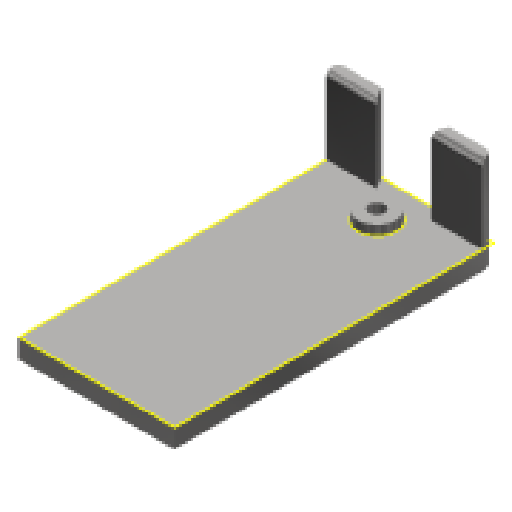
# Autodesk Inventor part: Gehäuse
Saved by Autodesk Inventor 2023 (Build 270158000, 158)
## iProperties
Created: 2025-01-24
Part Number: Gehäuse
Material: 1.2067 100 Cr 6 (WS)
Document SubType Name: Modeling
Designer: abdel
Density: 7.84 g/cm^3
Appearance: Stahl - poliert
Author: abdel
Autodesk Inventor part; units mm, degrees
ref_plane "YZ Plane" through (0, 0, 0) normal (1, 0, 0) x (0, 1, 0)
ref_plane "XZ Plane" through (0, 0, 0) normal (0, 1, 0) x (-1, 0, 0)
ref_plane "XY Plane" through (0, 0, 0) normal (0, 0, 1) x (1, 0, 0)
sketch "Skizze1" plane through (0, 0, 0) normal (0, 0, 1) x (1, 0, 0)
  line L0 (-20, 15) -> (20, 15)
  line L1 (20, 15) -> (20, -67)
  line L2 (20, -67) -> (-20, -67)
  line L3 (-20, -67) -> (-20, 15)
  line L4 (0, -83.4) -> (0, 31.4) projected
  point P0 (0, 0)
  point P1 (0, 15)
  dimension "d2" = 82
  dimension "d4" = 15
  dimension "d42" = 40
  constraints: 8 end point, 2 parallel, 1 horizontal, 1 midpoint, 1 perpendicular, 1 point on line
  measures "d2" distance of L2.end L0.start
  measures "d4" distance from line of point (0, 0) L0
  measures "d42" distance of L0.start L0.end
extrude "Extrusion1" add sketch "Skizze1" along normal blind 5
sketch "Skizze2" plane through (0, 0, 5) normal (0, 0, 1) x (1, 0, 0)
  line L0 (20, 15) -> (-20, 15) projected
  circle A0 centre (0, 5) radius 5
  line L1 (0, -83.4) -> (0, 31.4) projected
  point P0 (0, 0)
  dimension "d10" = 10
  dimension "d11" = 10
  constraints: 1 centre point, 1 point on line
  measures "d10" diameter of A0
  measures "d11" distance from line of A0.centre L0
extrude "Extrusion2" add sketch "Skizze2" along normal blind 2.5
sketch "Skizze3" plane through (0, 5, 7.5) normal (0, 0, 1) x (1, 0, 0)
  circle A0 centre (0, 0) radius 5 projected
  circle A1 centre (0, 0) radius 1
  point P0 (0, -5)
  dimension "d15" = 2
  constraints: 1 centre point, 1 coincident
  measures "d15" diameter of A1
hole "Bohrung1" at (0, 5, 7.5) direction (0, 0, -1) diameter 4 end through all
sketch "Skizze6" plane through (0, 0, 5) normal (0, 0, 1) x (1, 0, 0)
  line L0 (20, -67) -> (20, 15) projected
  line L1 (20, 15) -> (-20, 15) projected
  circle A0 centre (0, 5) radius 5 projected
  line L2 (-20, -67) -> (20, -67) projected
  line L3 (-20, 15) -> (-20, -67) projected
sketch "Skizze7" plane through (0, 0, 5) normal (0, 0, 1) x (1, 0, 0)
  circle A0 centre (0, 5) radius 5 projected
  line L0 (-20, -67) -> (20, -67) projected
  line L1 (20, -67) -> (20, 15) projected
  line L2 (20, 15) -> (-20, 15) projected
  line L3 (-20, 15) -> (-20, -67) projected
  point P0 (0, 0)
sketch "Skizze9" plane through (0, 0, 5) normal (0, 0, 1) x (1, 0, 0)
  line L0 (20, -67) -> (20, 15) projected
  line L1 (20, 15) -> (-20, 15) projected
  line L2 (-20, 15) -> (-20, -67) projected
  line L3 (20, 15) -> (20, 12)
  line L4 (20, 12) -> (-20, 12)
  line L5 (-20, 12) -> (-20, 15)
  line L6 (-8.7321, 15) -> (-7, 12)
  line L7 (8.7321, 15) -> (7, 12)
  line L8 (8.7321, 15) -> (12.1962, 15) construction
  line L9 (-20, 15) -> (-8.7321, 15)
  line L10 (8.7321, 15) -> (20, 15)
  point P0 (0, 0)
  point P1 (-8.7321, 15)
  dimension "d52" = 3
  dimension "d54" = 120
  dimension "d56" = 13
  dimension "d57" = 13
  dimension "d60" = 120
  constraints: 16 end point, 3 horizontal, 3 parallel, 3 point on line, 2 perpendicular, 1 collinear, 1 equal length
  measures "d52" distance between parallel lines of L4 L1
  measures "d54" angle of L7 L8
  measures "d56" distance from line of L0 L7.end
  measures "d57" distance from line of L2 L6.end
  measures "d60" angle of L4 L6
extrude "Extrusion6" add sketch "Skizze9" along normal blind 20 contours L4 L7 L1 L0 | L4 L2 L1 L6
fillet "Rundung1" radius 2 5 edges at (20, 15, 12.5) (-20, 15, 12.5) (0, 15, 0) (13.5, 12, 25) (-13.5, 12, 25)
